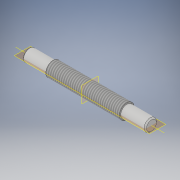
# Autodesk Inventor part: Large Gear Shaft
Saved by Autodesk Inventor 2019 (Build 230136000, 136)
## iProperties
Created: 2021-06-06
Part Number: Large Gear Shaft
Material: Generic
Document SubType Name: Modeling
Designer: micha
Density: 1 g/cm^3
Appearance: Default
Author: micha
Autodesk Inventor part; units mm, degrees
ref_plane "YZ Plane" through (0, 0, 0) normal (1, 0, 0) x (0, 1, 0)
ref_plane "XY Plane" through (0, 0, 0) normal (0, 0, 1) x (1, 0, 0)
sketch "Sketch1" plane through (0, 0, 0) normal (0, 0, 1) x (1, 0, 0)
  line L0 (0, 0) -> (60, 0)
  line L1 (60, 0) -> (60, 6)
  line L2 (60, 6) -> (0, 6)
  line L3 (0, 6) -> (0, 0)
  line L4 (0, 0) -> (0, 5)
  line L5 (0, 5) -> (-20, 5)
  line L6 (-20, 5) -> (-20, 0)
  line L7 (-20, 0) -> (0, 0)
  line L8 (60, 5) -> (80, 5)
  line L9 (80, 5) -> (80, 0)
  line L10 (80, 0) -> (60, 0)
  dimension "d0" = 60
  dimension "d1" = 6
  dimension "d3" = 5
  dimension "d4" = 20
  dimension "d5" = 20
  constraints: 22 end point, 7 perpendicular, 2 parallel, 2 point on line, 1 horizontal
  measures "d0" distance of L2.end L1.end
  measures "d1" distance of L1.end L0.end
  measures "d3" distance of L0.start L4.end
  measures "d4" distance of L4.end L5.end
  measures "d5" distance of L8.start L8.end
revolve "Revolution1" add sketch "Sketch1" angle 360 about axis through (0, 0, 0) along (1, 0, 0)
thread "Thread1" size "M12x1.75" class "6g" standard "ANSI Metric M Profile" full length
chamfer "Chamfer1" distance 1 angle 45 2 edges at (-20, -5, 0) (80, -5, 0)
ref_plane "Work Plane1" through (30, 0, 0) normal (1, 0, 0) x (0, 0, -1)
body "Solid1"
